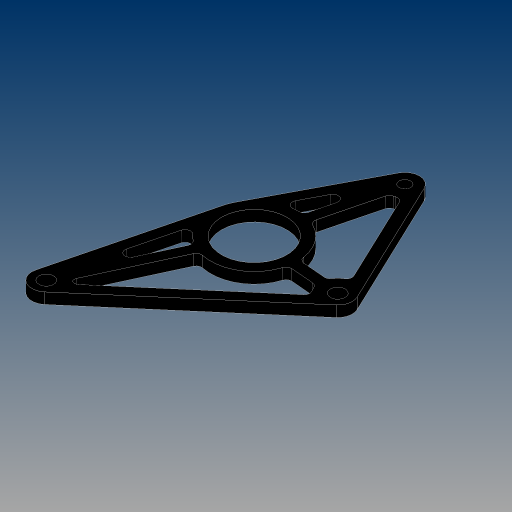
# Autodesk Inventor part: ELEV_036_SPRKTBRKT1
Saved by Autodesk Inventor 2024.3 (Build 283343000, 343)
## iProperties
Created: 2024-12-04
Part Number: ELEV_036_SPRKTBRKT1
Material: Aluminum 6061
Document SubType Name: Modeling
Designer: Kenji
Density: 2.7 g/cm^3
Appearance: Anodized - Black
Author: Kenji
Autodesk Inventor part; units mm, degrees
ref_plane "YZ Plane" through (0, 0, 0) normal (1, 0, 0) x (0, 1, 0)
ref_plane "XZ Plane" through (0, 0, 0) normal (0, 1, 0) x (-1, 0, 0)
ref_plane "XY Plane" through (0, 0, 0) normal (0, 0, 1) x (1, 0, 0)
sketch "Sketch1" plane through (0, 0, 0) normal (0, 1, 0) x (-1, 0, 0)
  circle A0 centre (0, 0) radius 14.2875
  line L0 (0, 0) -> (28.7924, 62.2152) construction
  line L1 (0, 0) -> (-39.9389, 3.3748) construction
  line L2 (0, 0) -> (-13.3336, -52.6166) construction
  circle A1 centre (28.7924, 62.2152) radius 3.2512
  circle A2 centre (-39.9389, 3.3748) radius 3.2512
  circle A3 centre (-13.3336, -52.6166) radius 2.54
  line L3 (0, 0) -> (0, 14.2875) construction
  circle A4 centre (28.7924, 62.2152) radius 6.35 construction
  circle A5 centre (-13.3336, -52.6166) radius 6.35 construction
  circle A6 centre (-39.9389, 3.3748) radius 6.35 construction
  circle A7 centre (0, 0) radius 19.05 construction
  line L4 (24.6628, 67.039) -> (-44.0685, 8.1986)
  line L5 (-45.6743, 0.6495) -> (-19.069, -55.3419)
  line L6 (16.8588, -8.8703) -> (-7.714, -55.5734)
  line L7 (18.4713, -4.6596) -> (34.9495, 60.662)
  arc A8 (34.9495, 60.662) -> (24.6628, 67.039) centre (28.7924, 62.2152) ccw
  arc A9 (-44.0685, 8.1986) -> (-45.6743, 0.6495) centre (-39.9389, 3.3748) ccw
  arc A10 (-19.069, -55.3419) -> (-7.714, -55.5734) centre (-13.3336, -52.6166) ccw
  arc A11 (16.8588, -8.8703) -> (18.4713, -4.6596) centre (0, 0) ccw
  dimension "d0" = 28.575
  dimension "d1" = 6.5024
  dimension "d2" = 68.5546
  dimension "d3" = 40.0812
  dimension "d4" = 54.2798
  dimension "d5" = 24.834
  dimension "d8" = 85.17
  dimension "d9" = 12.7
  dimension "d10" = 4.7625
  dimension "d32" = 80.61
  dimension "d33" = 5.08
  constraints: 16 end point, 16 point on circle, 11 centre point, 11 tangent, 8 coincident, 5 equal radius, 1 vertical, 1 vertical alignment, 2 other
  measures "d1" diameter of A1
  measures "d2" distance of L0.start L0.end
  measures "d3" distance of L0.start L1.end
  measures "d4" distance of L0.start L2.end
  measures "d5" angle of L3 L0
  measures "d8" angle of L1 L3
  measures "d9" diameter of A6
  measures "d32" angle of L1 L2
  measures "d33" diameter of A3
extrude "Extrusion1" add sketch "Sketch1" along normal blind 4.7625
sketch "Sketch2" plane through (0, 4.7625, 0) normal (0, 1, 0) x (1, 0, 0)
  line L0 (-18.4713, 4.6596) -> (-34.9495, -60.662) construction
  arc A0 (-34.9495, -60.662) -> (-24.6628, -67.039) centre (-28.7924, -62.2152) ccw construction
  line L1 (-24.6628, -67.039) -> (44.0685, -8.1986) construction
  arc A1 (44.0685, -8.1986) -> (45.6743, -0.6495) centre (39.9389, -3.3748) ccw construction
  line L2 (45.6743, -0.6495) -> (19.069, 55.3419) construction
  arc A2 (19.069, 55.3419) -> (7.714, 55.5734) centre (13.3336, 52.6166) ccw construction
  line L3 (7.714, 55.5734) -> (-16.8588, 8.8703) construction
  arc A3 (-16.8588, 8.8703) -> (-18.4713, 4.6596) centre (0, 0) ccw construction
  circle A4 centre (13.3336, 52.6166) radius 2.54 construction
  circle A5 centre (39.9389, -3.3748) radius 3.2512 construction
  circle A6 centre (-28.7924, -62.2152) radius 3.2512 construction
  circle A7 centre (0, 0) radius 14.2875 construction
  line L4 (-30.3316, -61.8269) -> (-13.8535, 3.4947) construction
  arc A8 (-12.6441, 6.6527) -> (-13.8535, 3.4947) centre (0, 0) ccw construction
  line L5 (-12.6441, 6.6527) -> (11.9287, 53.3558) construction
  arc A9 (14.7675, 53.298) -> (11.9287, 53.3558) centre (13.3336, 52.6166) ccw construction
  line L6 (14.7675, 53.298) -> (41.3727, -2.6935) construction
  arc A10 (40.9713, -4.5808) -> (41.3727, -2.6935) centre (39.9389, -3.3748) ccw construction
  line L7 (40.9713, -4.5808) -> (-27.76, -63.4212) construction
  arc A11 (-30.3316, -61.8269) -> (-27.76, -63.4212) centre (-28.7924, -62.2152) ccw construction
  circle A12 centre (-28.7924, -62.2152) radius 8.0137 construction
  circle A13 centre (0, 0) radius 19.05 construction
  circle A14 centre (39.9389, -3.3748) radius 8.0137 construction
  circle A15 centre (13.3336, 52.6166) radius 7.3025 construction
  line L8 (-25.4267, -54.9426) -> (-8.0008, -17.2884) construction
  line L9 (18.9824, -1.604) -> (31.9536, -2.7001) construction
  line L10 (4.6796, 18.4663) -> (11.5398, 45.5379) construction
  line L11 (-18.5688, -34.4995) -> (-10.9215, -17.975)
  line L12 (-22.7639, -54.8131) -> (-6.6339, -19.9592)
  line L13 (7.4237, 19.6791) -> (13.5496, 43.8526)
  line L14 (2.8441, 20.8396) -> (5.3686, 30.8015)
  line L15 (20.6266, -4.1136) -> (30.5232, -4.9498)
  line L16 (21.0244, 0.5941) -> (30.921, -0.2422)
  arc A16 (-3.9759, -18.6305) -> (18.1565, -5.7656) centre (0, 0) ccw
  arc A17 (-23.1205, -56.554) -> (-22.4788, -57.2797) centre (-28.7924, -62.2152) ccw
  arc A18 (32.5256, -6.4183) -> (33.4711, -8.1063) centre (39.9389, -3.3748) ccw
  line L17 (-19.8865, -56.6807) -> (33.0978, -11.3212)
  arc A19 (-22.7639, -54.8131) -> (-22.4788, -57.2797) centre (-20.6028, -55.8132) ccw
  arc A20 (-23.1205, -56.554) -> (-19.8865, -56.6807) centre (-21.4351, -54.8718) ccw
  arc A21 (-3.9759, -18.6305) -> (-6.6339, -19.9592) centre (-4.4729, -20.9593) ccw
  arc A22 (20.6266, -4.1136) -> (18.1565, -5.7656) centre (20.4261, -6.4864) ccw
  arc A23 (32.5256, -6.4183) -> (30.5232, -4.9498) centre (30.3227, -7.3226) ccw
  arc A24 (33.0978, -11.3212) -> (33.4711, -8.1063) centre (31.5492, -9.5123) ccw
  line L18 (36.9245, 6.668) -> (18.9095, 44.5809)
  arc A25 (18.8666, 2.6372) -> (8.6507, 16.9726) centre (0, 0) ccw
  arc A26 (15.2371, 45.5666) -> (15.9165, 45.7862) centre (13.3336, 52.6166) ccw
  arc A27 (35.9569, 3.5796) -> (33.1414, 0.8694) centre (39.9389, -3.3748) ccw
  arc A28 (7.4237, 19.6791) -> (8.6507, 16.9726) centre (9.732, 19.0941) ccw
  arc A29 (18.8666, 2.6372) -> (21.0244, 0.5941) centre (21.2249, 2.9669) ccw
  arc A30 (30.921, -0.2422) -> (33.1414, 0.8694) centre (31.1215, 2.1306) ccw
  arc A31 (35.9569, 3.5796) -> (36.9245, 6.668) centre (34.7737, 5.646) ccw
  arc A32 (15.2371, 45.5666) -> (13.5496, 43.8526) centre (15.8579, 43.2677) ccw
  arc A33 (18.9095, 44.5809) -> (15.9165, 45.7862) centre (16.7588, 43.5589) ccw
  line L19 (-4.3468, 22.4227) -> (0.9529, 32.4953)
  arc A34 (0.4763, 19.044) -> (-1.9906, 18.9457) centre (0, 0) ccw
  arc A35 (5.3686, 30.8015) -> (0.9529, 32.4953) centre (3.0603, 31.3865) ccw
  arc A36 (-4.3468, 22.4227) -> (-1.9906, 18.9457) centre (-2.2394, 21.3139) ccw
  arc A37 (0.4763, 19.044) -> (2.8441, 20.8396) centre (0.5358, 21.4246) ccw
  line L20 (-23.0388, -32.9169) -> (-18.2122, -13.7837)
  arc A38 (-14.1362, -12.7699) -> (-11.6289, -15.0888) centre (0, 0) ccw
  arc A39 (-23.0388, -32.9169) -> (-18.5688, -34.4995) centre (-20.7298, -33.4994) ccw
  arc A40 (-14.1362, -12.7699) -> (-18.2122, -13.7837) centre (-15.9033, -14.3661) ccw
  arc A41 (-10.9215, -17.975) -> (-11.6289, -15.0888) centre (-13.0825, -16.9749) ccw
  point P0 (-27.72, -54.2736)
  point P1 (-10.0829, -16.1629)
  point P2 (-23.4325, -56.2578)
  point P3 (-5.7953, -18.1471)
  point P4 (6.9333, 17.7435)
  point P5 (13.926, 45.3382)
  point P6 (2.3536, 18.904)
  point P7 (9.3464, 46.4987)
  point P8 (18.637, -3.9454)
  point P9 (32.1095, -5.0839)
  point P10 (19.0347, 0.7622)
  point P11 (32.5073, -0.3762)
  point P12 (-21.793, -58.3129)
  point P13 (35.0043, -9.689)
  point P14 (38.0016, 4.4012)
  point P15 (17.8266, 46.86)
  point P16 (-6.777, 17.8038)
  point P17 (8.6097, 47.0478)
  point P18 (-28.4103, -54.2106)
  point P19 (-16.9355, -8.7229)
  point P20 (-22.7397, -56.8639)
  dimension "d13" = 4.7625
  dimension "d14" = 4.7625
  dimension "d15" = 4.7625
  dimension "d16" = 4.7625
  dimension "d17" = 4.7625
  dimension "d18" = 2.3622
  dimension "d19" = 2.3622
  dimension "d20" = 2.3622
  dimension "d21" = 2.3622
  dimension "d22" = 2.3622
  dimension "d23" = 2.3622
  dimension "d24" = 2.3813
  dimension "d25" = 2.3813
  dimension "d26" = 2.3813
  dimension "d27" = 2.3813
  dimension "d28" = 2.3813
  dimension "d29" = 2.3813
  constraints: 90 point on circle, 36 tangent, 34 end point, 34 point on line, 33 centre point, 12 equal radius, 6 parallel, 4 concentric, 1 collinear, 25 other
  measures "d13" distance between parallel lines of L0 L4
  measures "d14" radial gap between concentric circles of A6 A12
  measures "d16" radial gap between concentric circles of A5 A14
  measures "d17" radial gap between concentric circles of A4 A15
  measures "d18" distance between parallel lines of L8 L11
  measures "d19" distance between parallel lines of L8 L12
  measures "d20" distance between parallel lines of L10 L13
  measures "d21" distance between parallel lines of L10 L14
  measures "d22" distance between parallel lines of L9 L15
  measures "d23" distance between parallel lines of L9 L16
  measures "d24" radius of A19
  measures "d25" radius of A28
  measures "d26" radius of A31
  measures "d27" radius of A33
  measures "d28" radius of A35
  measures "d29" radius of A39
extrude "Extrusion2" cut sketch "Sketch2" against normal blind 4.7625 contours A39 L20 A40 A38 A41 L11 | L12 A21 A16 A22 L15 A23 A18 A24 L17 A20 A19 | L13 A32 A26 A33 L18 A31 A27 A30 L16 A29 A25 A28 | A37 A34 A36 L19 A35 L14
body "Solid1"
